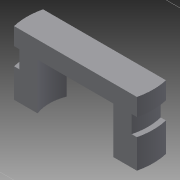
# Autodesk Inventor part: move male
Saved by Autodesk Inventor 2015 (Build 190159000, 159)
## iProperties
Created: 2018-12-22
Part Number: move male
Material: Типовые
Document SubType Name: Modeling
Designer: kostya
Density: 1 g/cm^3
Appearance: По умолчанию
Author: kostya
Autodesk Inventor part; units mm, degrees
ref_plane "YZ Plane" through (0, 0, 0) normal (1, 0, 0) x (0, 1, 0)
ref_plane "XZ Plane" through (0, 0, 0) normal (0, 1, 0) x (-1, 0, 0)
ref_plane "XY Plane" through (0, 0, 0) normal (0, 0, 1) x (1, 0, 0)
sketch "Эскиз1" plane through (0, 0, 0) normal (0, 0, 1) x (1, 0, 0)
  line L0 (-10.7121, -2.5) -> (10.5863, -2.5)
  line L1 (10.5863, 2.5) -> (-10.5863, 2.5)
  line L2 (-10.6663, -2.1333) -> (10.6663, 2.1333) construction
  line L3 (10.6663, -2.1333) -> (-10.6663, 2.1333) construction
  arc A0 (6.5383, -2.5) -> (6.5383, 2.5) centre (0, 0) ccw
  line L4 (0, 2.5) -> (0, -2.5) construction
  arc A1 (6.5383, -2.5) -> (6.5383, 2.5) centre (0, 0) ccw
  arc A2 (6.5383, -2.5) -> (6.5383, 2.5) centre (0, 0) ccw
  arc A3 (-6.5383, 2.5) -> (-6.5383, -2.5) centre (0, 0) ccw
  arc A4 (6.5383, -2.5) -> (6.5383, 2.5) centre (0, 0) ccw
  arc A5 (-9.6825, 2.5) -> (-9.6825, -2.5) centre (0, 0) ccw
  arc A6 (9.6825, -2.5) -> (9.6825, 2.5) centre (0, 0) ccw
  arc A7 (-10.5863, 2.5) -> (-10.5863, -2.5) centre (0, 0) ccw
  arc A8 (10.5863, -2.5) -> (10.5863, 2.5) centre (0, 0) ccw
  constraints: 22 point on circle, 10 end point, 10 point on line, 9 centre point, 3 midpoint, 2 coincident, 1 horizontal, 1 parallel
extrude "Выдавливание1" add sketch "Эскиз1" along normal blind 3
extrude "Выдавливание2" add sketch "Эскиз1" against normal blind 8 contours A7 L1 A5 L0 | A5 L1 A3 L0 | A0 L1 A6 L0 | A6 L1 A8 L0
extrude "Выдавливание3" cut sketch "Эскиз1" against normal blind 3 contours A7 L1 A5 L0 | A6 L1 A8 L0
